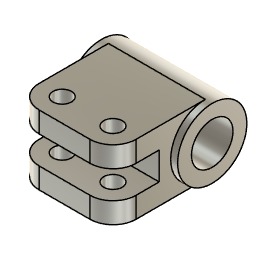
exercise10 (Autodesk Fusion 360 design; units mm, degrees)
Autodesk Fusion 360 part; units mm, degrees
note: some values were not read from the file. Set by a fixed rule: which sketch regions a step uses.
sketch "草图1" plane through (0, 0, 0) normal (1, 0, 0) x (0, 1, 0)
  circle A0 centre (0, 0) radius 15
  circle A1 centre (0, 0) radius 9
  line L0 (0, 15) -> (-40, 15)
  line L1 (-40, 15) -> (-40, 6)
  line L2 (-40, 6) -> (-20, 6)
  line L3 (-20, 6) -> (-20, -6)
  line L4 (-20, -6) -> (-40, -6)
  line L5 (-40, -6) -> (-40, -15)
  line L6 (-40, -15) -> (0, -15)
  line L7 (-157.7005, 0) -> (55, 0) construction
  dimension "d1" = 30
  dimension "d2" = 18
  dimension "d3" = 12
  dimension "d4" = 20
  dimension "d5" = 40
  constraint coincident A0.centre A1.centre
  constraint concentric A0 A1
  constraint perpendicular L1 L2
  constraint perpendicular L2 L3
  constraint horizontal L4
  constraint parallel L4 L7
  constraint symmetric L0 L6 L7
  constraint parallel L0 L7
  constraint parallel L2 L6
  constraint perpendicular L4 L5
  constraint symmetric L2 L4 L7
  constraint tangent A0 L0
  constraint equal L2 L4
  constraint coincident A0 L0.start
  constraint coincident A0 L6.end
  measures "d1" diameter of A0
  measures "d2" diameter of A1
  measures "d3" distance of L2.end L3.end
  measures "d4" horizontal distance of A0.centre L2.end
  measures "d5" distance of A0.centre L1
extrude "拉伸1" add sketch "草图1" along normal mid plane 48 contours A0
extrude "拉伸2" add sketch "草图1" along normal mid plane 42 contours A0 L0 L1 L2 L3 L4 L5 L6
fillet "圆角1" radius 10 4 edges at (21, -40, 10.5) (21, -40, -10.5) (-21, -40, 10.5) (-21, -40, -10.5)
sketch "草图2" plane through (0, 0, 15) normal (0, 0, 1) x (-1, 0, 0)
  arc A0 (21, 30) -> (11, 40) centre (11, 30) ccw
  line L0 (11, 40) -> (-11, 40)
  arc A1 (-11, 40) -> (-21, 30) centre (-11, 30) ccw
  line L1 (-21, 30) -> (-21, 0)
  line L2 (-21, 0) -> (21, 0)
  line L3 (21, 0) -> (21, 30)
  line L4 (21, 30) -> (-21, 30)
  circle A2 centre (11, 30) radius 4
  circle A3 centre (-11, 30) radius 4
  line L5 (0, 0) -> (0, 40)
  line L6 (-11, 30) -> (-11, 40)
  dimension "d12" = 8
  constraint coincident A0.start L3.end
  constraint coincident A1.end L1.start
  constraint coincident L4 A0.centre
  constraint concentric A1 A3
  constraint symmetric A2 A3 L5
  constraint coincident A1.centre A3.centre
  constraint coincident L0.end A1.start
  measures "d12" diameter of A2
extrude "拉伸3" cut sketch "草图2" against normal through all contours L4 A2 | L4 A2 | L4 A3 L6 | L4 A3 L6 | L4 A3
